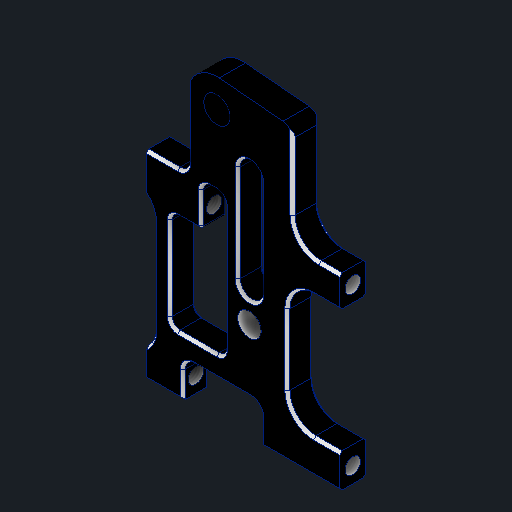
# Autodesk Inventor part: Z25_Sideplate
Saved by Autodesk Inventor 2025 (Build 290162010, 162A)
## iProperties
Created: 2023-02-03
Part Number: Z25_Sideplate
Material: Aluminum 6061
Document SubType Name: Modeling
Designer: dzw04
Density: 2.7 g/cm^3
Appearance: Aluminum - Flat
Author: dzw04
Autodesk Inventor part; units mm, degrees
ref_plane "YZ Plane" through (0, 0, 0) normal (1, 0, 0) x (0, 1, 0)
ref_plane "XZ Plane" through (0, 0, 0) normal (0, 1, 0) x (-1, 0, 0)
ref_plane "XY Plane" through (0, 0, 0) normal (0, 0, 1) x (1, 0, 0)
sketch "Sketch1" plane through (0, 0, 0) normal (0, 0, 1) x (1, 0, 0)
  circle A0 centre (13.5, 51.5) radius 2.5
  circle A1 centre (19.75, 19) radius 1.5
  line L0 (26.1743, 55.9122) -> (13.9794, 56.9791)
  arc A2 (13.9794, 56.9791) -> (8, 51.5) centre (13.5, 51.5) ccw
  line L1 (8, 51.5) -> (8, 40)
  arc A3 (6, 38) -> (8, 40) centre (6, 40) ccw
  line L2 (6, 38) -> (0, 38)
  line L3 (0, 38) -> (0, 30.5)
  arc A4 (1.5, 26.9293) -> (0, 30.5) centre (-3.5, 26.9293) ccw
  line L4 (1.5, 26.9293) -> (1.5, 9.0707)
  arc A5 (0, 5.5) -> (1.5, 9.0707) centre (-3.5, 9.0707) ccw
  line L5 (0, 5.5) -> (0, 0)
  line L6 (0, 0) -> (7, 0)
  line L7 (7, 0) -> (7, 5)
  arc A6 (9, 7) -> (7, 5) centre (9, 5) ccw
  line L8 (9, 7) -> (20, 7)
  arc A7 (22, 5) -> (20, 7) centre (20, 5) ccw
  line L9 (22, 5) -> (22, 0)
  line L10 (22, 0) -> (37, 0)
  line L11 (37, 0) -> (37, 6.5)
  line L12 (37, 6.5) -> (32, 6.5)
  arc A8 (27, 11.5) -> (32, 6.5) centre (32, 11.5) ccw
  line L13 (27, 11.5) -> (27, 25)
  arc A9 (32, 30) -> (27, 25) centre (32, 25) ccw
  line L14 (32, 30) -> (37, 30)
  line L15 (37, 30) -> (37, 36)
  line L16 (37, 36) -> (33, 36)
  arc A10 (28, 41) -> (33, 36) centre (33, 41) ccw
  line L17 (28, 41) -> (28, 53.9198)
  arc A11 (28, 53.9198) -> (26.1743, 55.9122) centre (26, 53.9198) ccw
  line L18 (4.5, 12.5) -> (4.5, 28.5)
  arc A12 (6, 30) -> (4.5, 28.5) centre (6, 28.5) ccw
  line L19 (6, 30) -> (10, 30)
  arc A13 (10, 30) -> (10.5, 30.5) centre (10, 30.5) ccw
  line L20 (10.5, 30.5) -> (10.5, 36.5)
  arc A14 (12, 38) -> (10.5, 36.5) centre (12, 36.5) ccw
  line L21 (12, 38) -> (13.5, 38)
  arc A15 (15, 36.5) -> (13.5, 38) centre (13.5, 36.5) ccw
  line L22 (15, 36.5) -> (15, 12.5)
  arc A16 (13.5, 11) -> (15, 12.5) centre (13.5, 12.5) ccw
  line L23 (13.5, 11) -> (6, 11)
  arc A17 (4.5, 12.5) -> (6, 11) centre (6, 12.5) ccw
  line L24 (17.5, 43.75) -> (17.5, 25.25)
  arc A18 (17.5, 25.25) -> (22, 25.25) centre (19.75, 25.25) ccw
  line L25 (22, 25.25) -> (22, 43.75)
  arc A19 (22, 43.75) -> (17.5, 43.75) centre (19.75, 43.75) ccw
  point P0 (8, 51.5)
  point P1 (0, 5.5)
  point P2 (9, 7)
  point P3 (27, 11.5)
  constraints: 52 end point, 36 point on circle, 20 centre point
extrude "Extrusion1" add sketch "Sketch1" along normal blind 5
chamfer "Chamfer1" distance 0.5 angle 45 62 edges at (1.5, 18, 5) (1.1098, 7.1342, 5) (1.1098, 28.8658, 5) (1.5, 18, 0) (1.1098, 7.1342, 0) (1.1098, 28.8658, 0) (15, 24.5, 5) (14.5607, 11.4393, 5) (9.75, 11, 5) (4.9393, 11.4393, 5) (4.5, 20.5, 5) (4.9393, 29.5607, 5) (8, 30, 5) (10.3536, 30.1464, 5) (10.5, 33.5, 5) (10.9393, 37.5607, 5) (12.75, 38, 5) (14.5607, 37.5607, 5) (15, 24.5, 0) (14.5607, 11.4393, 0) (9.75, 11, 0) (4.9393, 11.4393, 0) (4.5, 20.5, 0) (4.9393, 29.5607, 0) (8, 30, 0) (10.3536, 30.1464, 0) (10.5, 33.5, 0) (10.9393, 37.5607, 0) (12.75, 38, 0) (14.5607, 37.5607, 0) (17.5, 34.5, 5) (19.75, 46, 5) (22, 34.5, 5) (19.75, 23, 5) (22, 34.5, 0) (19.75, 23, 0) (17.5, 34.5, 0) (19.75, 46, 0) (14.5, 7, 5) (21.4142, 6.4142, 5) (22, 2.5, 5) (7.5858, 6.4142, 5) (7, 2.5, 5) (14.5, 7, 0) (21.4142, 6.4142, 0) (22, 2.5, 0) (7.5858, 6.4142, 0) (7, 2.5, 0) (29.5, 0, 5) (29.5, 0, 0) (3.5, 0, 5) (3.5, 0, 0) (27, 18.25, 5) (28.4645, 28.5355, 5) (34.5, 30, 5) (28.4645, 7.9645, 5) (34.5, 6.5, 5) (27, 18.25, 0) (28.4645, 28.5355, 0) (34.5, 30, 0) (28.4645, 7.9645, 0) (34.5, 6.5, 0)
chamfer "Chamfer2" distance 0.5 angle 45 12 edges at (3, 38, 5) (7.4142, 38.5858, 5) (8, 45.75, 5) (28, 47.4599, 5) (29.4645, 37.4645, 5) (35, 36, 5) (29.4645, 37.4645, 0) (35, 36, 0) (28, 47.4599, 0) (8, 45.75, 0) (7.4142, 38.5858, 0) (3, 38, 0)
sketch "Sketch2" plane through (37, 30, 4.5) normal (1, 0, 0) x (0, 0, -1)
  line L0 (4, 6) -> (4.5, 5.5) projected
  line L1 (4, 6) -> (0, 6) projected
  line L2 (-0.5, 5.5) -> (0, 6) projected
  line L3 (-0.5, 0.5) -> (-0.5, 5.5) projected
  line L4 (0, 0) -> (-0.5, 0.5) projected
  line L5 (4, 0) -> (0, 0) projected
  line L6 (4.5, 0.5) -> (4, 0) projected
  line L7 (4.5, 0.5) -> (4.5, 5.5) projected
  line L8 (4, -23.5) -> (4.5, -24) projected
  line L9 (4, -23.5) -> (0, -23.5) projected
  line L10 (-0.5, -24) -> (0, -23.5) projected
  line L11 (-0.5, -29.5) -> (-0.5, -24) projected
  line L12 (0, -30) -> (-0.5, -29.5) projected
  line L13 (4, -30) -> (0, -30) projected
  line L14 (4.5, -29.5) -> (4, -30) projected
  line L15 (4.5, -29.5) -> (4.5, -24) projected
  line L16 (-0.5, 0.5) -> (-0.5, 5.5) projected
  line L17 (-0.5, 3) -> (4.5, 3) construction
  line L18 (4.5, 0.5) -> (4.5, 5.5) projected
  circle A0 centre (2, 3) radius 1.5
  line L19 (2, 3) -> (2, -27) construction
  line L20 (4, -30) -> (0, -30) projected
  circle A1 centre (2, -27) radius 1.5
  point P0 (4.5, -30)
  dimension "d8" = 3
  dimension "d9" = 30
  dimension "d10" = 3
  constraints: 4 end point, 3 midpoint, 2 centre point, 1 coincident, 1 perpendicular
  measures "d8" diameter of A0
  measures "d9" distance of L19.start L19.end
  measures "d10" diameter of A1
extrude "Extrusion2" cut sketch "Sketch2" against normal up to surface (15 mm away) contours A0 | A1
sketch "Sketch3" plane through (0, 0.5, 0) normal (-1, 0, 0) x (0, 0, 1)
  circle A0 centre (2.5, 2.5) radius 1.5 projected
  circle A1 centre (2.5, 2.5) radius 1.5 projected
  circle A2 centre (2.5, 32.5) radius 1.5 projected
  point P0 (0, -0.5)
extrude "Extrusion3" cut sketch "Sketch3" against normal up to surface (10.5 mm away)
thread "Thread1" size "M3x0.5" class "6H" standard "ANSI Metric M Profile" full length
thread "Thread2" size "M3x0.5" class "6H" standard "ANSI Metric M Profile" full length
thread "Thread3" size "M3x0.5" class "6H" standard "ANSI Metric M Profile" full length
thread "Thread4" size "M3x0.5" class "6H" standard "ANSI Metric M Profile" full length
sketch "Sketch4" plane through (0, 0, 5) normal (0, 0, 1) x (1, 0, 0)
  circle A0 centre (19.75, 19) radius 1.5 projected
  circle A1 centre (19.75, 19) radius 2.25
  point P0 (0, 0)
  dimension "d23" = 4.5
  constraints: 1 centre point, 1 coincident
  measures "d23" diameter of A1
extrude "Extrusion4" cut sketch "Sketch4" against normal through all
equation "\"d11\" = d8"
body "Solid1"
